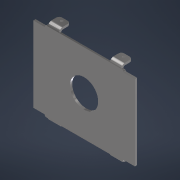
# Autodesk Inventor part: BaseSistema
Saved by Autodesk Inventor 2022 (Build 260153000, 153)
## iProperties
Created: 2021-09-29
Part Number: BaseSistema
Material: Steel, Alloy
Document SubType Name: Sheet Metal
Designer: Andres
Density: 7.73 g/cm^3
Sheet Metal Rule: Default_mm
Appearance: Semi-Polished
Author: Andres
Autodesk Inventor part; units mm, degrees
ref_plane "YZ Plane" through (0, 0, 0) normal (1, 0, 0) x (0, 1, 0)
ref_plane "XZ Plane" through (0, 0, 0) normal (0, 1, 0) x (-1, 0, 0)
ref_plane "XY Plane" through (0, 0, 0) normal (0, 0, 1) x (1, 0, 0)
sketch "Sketch1" plane through (0, 0, 0) normal (0, 0, 1) x (1, 0, 0)
  arc A0 (-67, 70) -> (-70, 67) centre (-67, 67) ccw projected
  line L0 (-70, 67) -> (-70, -67) projected
  arc A1 (-70, -67) -> (-67, -70) centre (-67, -67) ccw projected
  line L1 (-67, -70) -> (67, -70) projected
  arc A2 (67, -70) -> (70, -67) centre (67, -67) ccw projected
  line L2 (70, -67) -> (70, 67) projected
  arc A3 (70, 67) -> (67, 70) centre (67, 67) ccw projected
  line L3 (67, 70) -> (-67, 70) projected
  circle A4 centre (0, 0) radius 27 projected
  line L4 (65, 90) -> (45, 90)
  line L5 (45, 90) -> (45, 70)
  line L6 (70, 0) -> (-70, 0) construction
  line L7 (90, 67) -> (90, -67)
  line L8 (-90, 67) -> (-90, -67)
  line L9 (65, 70) -> (65, 90)
  line L10 (-90, -67) -> (-70, -67)
  line L11 (-70, 67) -> (-90, 67)
  line L12 (90, 67) -> (70, 67)
  line L13 (70, -67) -> (90, -67)
  line L14 (0, 70) -> (0, -70) construction
  line L15 (-65, 90) -> (-45, 90)
  line L16 (-45, 90) -> (-45, 70)
  line L17 (-65, 70) -> (-65, 90)
  line L18 (65, -90) -> (45, -90)
  line L19 (45, -90) -> (45, -70)
  line L20 (65, -70) -> (65, -90)
  line L21 (-45, -90) -> (-45, -70)
  line L22 (-65, -90) -> (-45, -90)
  line L23 (-65, -70) -> (-65, -90)
  line L24 (55, 90) -> (55, 70) construction
  line L25 (-55, 90) -> (-55, 70) construction
  line L26 (-45, 70) -> (-65, 70)
  line L27 (-45, -70) -> (-65, -70)
  line L28 (65, -70) -> (45, -70)
  line L29 (65, 70) -> (45, 70)
  line L30 (45, 70) -> (45, 68)
  line L31 (45, 68) -> (65, 68)
  line L32 (65, 68) -> (65, 70)
  line L33 (45, -70) -> (45, -68)
  line L34 (45, -68) -> (65, -68)
  line L35 (65, -68) -> (65, -70)
  line L36 (-45, -70) -> (-45, -68)
  line L37 (-45, -68) -> (-65, -68)
  line L38 (-65, -68) -> (-65, -70)
  line L39 (-65, 70) -> (-65, 68)
  line L40 (-65, 68) -> (-45, 68)
  line L41 (-45, 68) -> (-45, 70)
  line L42 (65, 68) -> (69.8284, 68)
  dimension "d1" = 20
  dimension "d4" = 20
  dimension "d26" = 110
  dimension "d27" = 20
  dimension "d37" = 2
  dimension "d38" = 2
  dimension "d39" = 2
  dimension "d40" = 2
  constraints: 79 end point, 15 perpendicular, 12 symmetric about line, 6 midpoint, 6 vertical, 5 collinear, 4 point on line, 2 horizontal, 1 point on circle
  measures "d1" distance of L4.start L4.end
  measures "d4" distance between parallel lines of L2 L7
  measures "d26" distance between parallel lines of L25 L24
  measures "d27" distance between parallel lines of L3 L4
  measures "d37" distance between parallel lines of L29 L31
  measures "d38" distance between parallel lines of L28 L34
  measures "d39" distance between parallel lines of L1 L37
  measures "d40" distance between parallel lines of L40 L3
extrude "Plate1" add sketch "Sketch1" along normal blind 4 contours L3 L39 L40 L41 L30 L31 L42 A3 L2 A2 L1 L35 L34 L33 L36 L37 L38 A1 L0 A0 | L0 L10 L8 L11 | L17 L15 L16 L3 | L3 L41 L40 L39 | L5 L4 L9 L3 | L3 L32 L31 L30 | L38 L37 L36 L1 | L1 L21 L22 L23 | L3 A3 L42 L32 | L33 L34 L35 L1 | L1 L20 L18 L19 | L12 L7 L13 L2 | A4
sketch "Sketch3" plane through (0, 0, 0) normal (0, 0, -1) x (-1, 0, 0)
  line L0 (-90, 67) -> (-70, 67) projected
  line L1 (-90, -67) -> (-90, 67) projected
  line L2 (-70, -67) -> (-90, -67) projected
  arc A0 (-70, -67) -> (-67, -70) centre (-67, -67) ccw projected
  line L3 (-65, -70) -> (-67, -70) projected
  line L4 (-65, -90) -> (-65, -70) projected
  line L5 (-45, -90) -> (-65, -90) projected
  line L6 (-45, -70) -> (-45, -90) projected
  line L7 (45, -70) -> (-45, -70) projected
  line L8 (45, -70) -> (45, -90) projected
  line L9 (45, -90) -> (65, -90) projected
  line L10 (65, -90) -> (65, -70) projected
  line L11 (67, -70) -> (65, -70) projected
  arc A1 (67, -70) -> (70, -67) centre (67, -67) ccw projected
  line L12 (90, -67) -> (70, -67) projected
  line L13 (90, 67) -> (90, -67) projected
  line L14 (70, 67) -> (90, 67) projected
  arc A2 (70, 67) -> (67, 70) centre (67, 67) ccw projected
  line L15 (65, 70) -> (67, 70) projected
  line L16 (65, 90) -> (65, 70) projected
  line L17 (45, 90) -> (65, 90) projected
  line L18 (45, 70) -> (45, 90) projected
  line L19 (-45, 70) -> (45, 70) projected
  line L20 (-45, 90) -> (-45, 70) projected
  line L21 (-65, 90) -> (-45, 90) projected
  line L22 (-65, 70) -> (-65, 90) projected
  line L23 (-67, 70) -> (-65, 70) projected
  arc A3 (-67, 70) -> (-70, 67) centre (-67, 67) ccw projected
  line L24 (69.8284, 68) -> (-69.8284, 68)
  line L25 (-45, 70) -> (45, 70) projected
  line L26 (69.8284, -68) -> (-69.8284, -68)
  line L27 (45, -70) -> (-45, -70) projected
  point P0 (0, 0)
  dimension "d41" = 2
  dimension "d48" = 2
  constraints: 4 end point, 4 point on circle, 2 parallel
  measures "d41" distance between parallel lines of L24 L19
  measures "d48" distance between parallel lines of L26 L7
fold "Fold4" angle 90 bend radius 4 thickness 4 k factor 0.44 line from (-69.8284, 68, 0) to (69.8284, 68, 0) line at bend start moving side (0, 1, 0) folds toward (0, 0, -1)
fold "Fold5" angle 90 bend radius 4 thickness 4 k factor 0.44 line from (-69.8284, -68, 0) to (69.8284, -68, 0) line at bend start moving side (0, -1, 0) folds toward (0, 0, -1)
fillet "Corner Round1" radius 5 8 edges at (65, 74, -16.9522) (45, 74, -16.9522) (65, -74, -16.9522) (45, -74, -16.9522) (-45, -74, -16.9522) (-65, -74, -16.9522) (-65, 74, -16.9522) (-45, 74, -16.9522)
sketch "Sketch4" plane through (45, -76, -4) normal (0, -1, 0) x (1, 0, 0)
  arc A0 (0, -7.9522) -> (5, -12.9522) centre (5, -7.9522) ccw projected
  line L0 (15, -12.9522) -> (5, -12.9522) projected
  arc A1 (15, -12.9522) -> (20, -7.9522) centre (15, -7.9522) ccw projected
  line L1 (20, 0) -> (20, -7.9522) projected
  line L2 (20, 0) -> (0, 0) projected
  line L3 (0, -7.9522) -> (0, 0) projected
  arc A2 (-110, -7.9522) -> (-105, -12.9522) centre (-105, -7.9522) ccw projected
  line L4 (-95, -12.9522) -> (-105, -12.9522) projected
  arc A3 (-95, -12.9522) -> (-90, -7.9522) centre (-95, -7.9522) ccw projected
  line L5 (-90, 0) -> (-90, -7.9522) projected
  line L6 (-90, 0) -> (-110, 0) projected
  line L7 (-110, -7.9522) -> (-110, 0) projected
  line L8 (-110, 3.7613) -> (-112, 3.7613) projected
  line L9 (24.8284, 4) -> (-114.8284, 4) projected
  line L10 (-115, 4) -> (-114.8284, 4) projected
  line L11 (-135, 4) -> (-115, 4) projected
  line L12 (-115, 4) -> (-135, 4) projected
  line L13 (-114.8284, 4) -> (-115, 4) projected
  line L14 (-114.8284, 4) -> (24.8284, 4) projected
  line L15 (25, 4) -> (24.8284, 4) projected
  line L16 (45, 4) -> (25, 4) projected
  line L17 (25, 4) -> (45, 4) projected
  line L18 (24.8284, 4) -> (25, 4) projected
  point P0 (-45, 4)
  point P1 (10, -7.5)
  point P2 (-100, -7.5)
  point P3 (10, -12.9522)
  point P4 (-100, -12.9522)
  point P5 (0, 1.5368)
  point P6 (-90, 1.5368)
  point P7 (-110, 1.5368)
  point P8 (-112, 1.5368)
  point P9 (-110, 2.6842)
  point P10 (-112, 2.6842)
  point P11 (-110, 4.8083)
  point P12 (-112, 4.8083)
  dimension "d63" = 11.5
  constraints: 2 midpoint, 2 vertical alignment, 1 horizontal alignment, 1 other
  measures "d63" distance from line of point (-100, -7.5) L11
hole "Hole2" at (55, -76, -11.5) at (-55, -76, -11.5) direction (0, 1, 0) diameter 4.5 end through all clearance for "Hex Head Cap Screw ISO 24014 (Spotface)" size "M4" standard "ISO"
sketch "Sketch5" plane through (0, 0, 0) normal (0, 0, -1) x (-1, 0, 0)
  circle A0 centre (0, 0) radius 25
  dimension "d64" = 50
  constraints: 1 centre point, 1 coincident
  measures "d64" diameter of A0
extrude "Cut1" cut sketch "Sketch5" against normal blind 4
equation "\"d38\" = d37"
equation "\"d39\" = d37"
equation "\"d40\" = d37"
equation "\"d48\" = d41"
equation "\"d5\" = Thickness"
equation "\"d42\" = BendReliefWidth"
equation "\"d43\" = BendReliefDepth"
equation "\"d44\" = MinimumRemnant"
equation "\"d45\" = TransitionRadius"
equation "\"d47\" = BendRadius"
equation "\"d49\" = BendReliefWidth"
equation "\"d50\" = BendReliefDepth"
equation "\"d51\" = MinimumRemnant"
equation "\"d52\" = TransitionRadius"
equation "\"d54\" = BendRadius"
equation "\"d61\" = Thickness"
equation "\"d65\" = Thickness"
equation "\"BendRadius\" = Thickness"
equation "\"BendReliefWidth\" = Thickness"
equation "\"BendReliefDepth\" = 0.5 * Thickness"
equation "\"CornerReliefSize\" = 4 * Thickness"
equation "\"MinimumRemnant\" = 2 * Thickness"
equation "\"TransitionRadius\" = BendRadius"
equation "\"JacobiRadiusSize\" = BendRadius"
equation "\"GapSize\" = Thickness"
equation "\"Thickness\" = 4"
body "Solid2"
